Autodesk Fusion 360 part; units mm, degrees
(part 7 of 8)
  spline S19 degree 5 poles (-0.8149, 14.5372) (-0.8168, 14.5341) (-0.8204, 14.528) (-0.8258, 14.5188) (-0.833, 14.5066) (-0.842, 14.4913) (-0.8509, 14.4761) (-0.8597, 14.4608) (-0.8685, 14.4456) (-0.8773, 14.4304) (-0.886, 14.4152) (-0.8946, 14.4) (-0.9032, 14.3848) (-0.9117, 14.3697) (-0.9202, 14.3545) (-0.9286, 14.3394) (-0.937, 14.3243) (-0.9453, 14.3092) (-0.9536, 14.2941) (-0.9618, 14.2791) (-0.97, 14.264) (-0.9781, 14.249) (-0.9862, 14.234) (-0.9942, 14.219) (-1.0021, 14.204) (-1.01, 14.189) (-1.0179, 14.1741) (-1.0257, 14.1592) (-1.0334, 14.1443) (-1.0411, 14.1294) (-1.0488, 14.1145) (-1.0564, 14.0996) (-1.0639, 14.0848) (-1.0714, 14.07) (-1.0788, 14.0552) (-1.0862, 14.0404) (-1.0935, 14.0257) (-1.1008, 14.0109) (-1.108, 13.9962) (-1.1152, 13.9815) (-1.1223, 13.9669) (-1.1294, 13.9522) (-1.1364, 13.9376) (-1.1434, 13.923) (-1.1503, 13.9084) (-1.1572, 13.8938) (-1.164, 13.8793) (-1.1707, 13.8648) (-1.1775, 13.8503) (-1.1841, 13.8358) (-1.1907, 13.8214) (-1.1973, 13.807) (-1.2038, 13.7926) (-1.2102, 13.7782) (-1.2166, 13.7639) (-1.223, 13.7495) (-1.2293, 13.7352) (-1.2355, 13.721) (-1.2417, 13.7067) (-1.2478, 13.6925) (-1.2539, 13.6783) (-1.26, 13.6642) (-1.266, 13.65) (-1.2719, 13.6359) (-1.2778, 13.6218) (-1.2836, 13.6078) (-1.2894, 13.5938) (-1.2951, 13.5798) (-1.3008, 13.5658) (-1.3064, 13.5519) (-1.312, 13.538) (-1.3176, 13.5241) (-1.323, 13.5103) (-1.3285, 13.4964) (-1.3338, 13.4827) (-1.3392, 13.4689) (-1.3444, 13.4552) (-1.3497, 13.4415) (-1.3548, 13.4279) (-1.36, 13.4142) (-1.3651, 13.4006) (-1.3701, 13.3871) (-1.3751, 13.3736) (-1.38, 13.3601) (-1.3849, 13.3466) (-1.3897, 13.3332) (-1.3945, 13.3198) (-1.3992, 13.3065) (-1.4039, 13.2932) (-1.4085, 13.2799) (-1.4131, 13.2666) (-1.4176, 13.2534) (-1.4221, 13.2403) (-1.4265, 13.2271) (-1.4309, 13.214) (-1.4353, 13.201) (-1.4396, 13.188) (-1.4438, 13.175) (-1.448, 13.162) (-1.4521, 13.1491) (-1.4562, 13.1363) (-1.4603, 13.1235) (-1.4643, 13.1107) (-1.4682, 13.0979) (-1.4721, 13.0852) (-1.476, 13.0726) (-1.4798, 13.06) (-1.4835, 13.0474) (-1.4872, 13.0349) (-1.4909, 13.0224) (-1.4945, 13.01) (-1.4981, 12.9976) (-1.5016, 12.9852) (-1.5051, 12.9729) (-1.5085, 12.9606) (-1.5119, 12.9484) (-1.5152, 12.9362) (-1.5185, 12.9241) (-1.5218, 12.912) (-1.5249, 12.9) (-1.5281, 12.888) (-1.5312, 12.8761) (-1.5343, 12.8642) (-1.5373, 12.8524) (-1.5402, 12.8406) (-1.5432, 12.8288) (-1.546, 12.8171) (-1.5489, 12.8055) (-1.5517, 12.7939) (-1.5544, 12.7824) (-1.5571, 12.7709) (-1.5597, 12.7595) (-1.5624, 12.7481) (-1.5649, 12.7368) (-1.5674, 12.7255) (-1.5699, 12.7143) (-1.5723, 12.7031) (-1.5747, 12.692) (-1.5771, 12.681) (-1.5794, 12.67) (-1.5816, 12.659) (-1.5839, 12.6482) (-1.586, 12.6373) (-1.5882, 12.6266) (-1.5903, 12.6159) (-1.5923, 12.6052) (-1.5943, 12.5946) (-1.5963, 12.5841) (-1.5982, 12.5736) (-1.6001, 12.5632) (-1.6019, 12.5529) (-1.6037, 12.5426) (-1.6055, 12.5324) (-1.6072, 12.5223) (-1.6089, 12.5122) (-1.6105, 12.5022) (-1.6121, 12.4922) (-1.6137, 12.4823) (-1.6152, 12.4725) (-1.6167, 12.4627) (-1.6182, 12.453) (-1.6196, 12.4434) (-1.6209, 12.4339) (-1.6223, 12.4244) (-1.6236, 12.415) (-1.6248, 12.4056) (-1.626, 12.3964) (-1.6272, 12.3872) (-1.6284, 12.3781) (-1.6295, 12.369) (-1.6306, 12.36) (-1.6316, 12.3511) (-1.6326, 12.3423) (-1.6336, 12.3336) (-1.6345, 12.3249) (-1.6354, 12.3163) (-1.6363, 12.3078) (-1.6371, 12.2994) (-1.6379, 12.291) (-1.6387, 12.2827) (-1.6394, 12.2746) (-1.6401, 12.2665) (-1.6408, 12.2584) (-1.6414, 12.2505) (-1.6421, 12.2426) (-1.6426, 12.2349) (-1.6432, 12.2272) (-1.6437, 12.2196) (-1.6442, 12.2121) (-1.6447, 12.2047) (-1.6451, 12.1974) (-1.6455, 12.1901) (-1.6459, 12.183) (-1.6462, 12.1759) (-1.6466, 12.169) (-1.6469, 12.1621) (-1.6471, 12.1554) (-1.6474, 12.1487) (-1.6476, 12.1421) (-1.6478, 12.1357) (-1.648, 12.1293) (-1.6481, 12.123) (-1.6483, 12.1169) (-1.6484, 12.1108) (-1.6484, 12.1048) (-1.6485, 12.099) (-1.6486, 12.0933) (-1.6486, 12.0876) (-1.6486, 12.0821) (-1.6486, 12.0767) (-1.6486, 12.0714) (-1.6485, 12.0662) (-1.6485, 12.0611) (-1.6484, 12.0562) (-1.6483, 12.0514) (-1.6482, 12.0466) (-1.6481, 12.042) (-1.6479, 12.0376) (-1.6478, 12.0332) (-1.6476, 12.029) (-1.6475, 12.0249) (-1.6473, 12.021) (-1.6471, 12.0171) (-1.6469, 12.0134) (-1.6468, 12.0099) (-1.6466, 12.0064) (-1.6464, 12.0031) (-1.6462, 12) (-1.646, 11.997) (-1.6457, 11.9941) (-1.6455, 11.9914) (-1.6453, 11.9889) (-1.6451, 11.9865) (-1.6449, 11.9842) (-1.6448, 11.9821) (-1.6446, 11.9802) (-1.6444, 11.9784) (-1.6442, 11.9768) (-1.6441, 11.9753) (-1.6439, 11.974) (-1.6438, 11.9729) (-1.6437, 11.9722) (-1.6437, 11.9717) (-1.6436, 11.9714) (-1.6436, 11.9713) knots -1 -1 -1 -1 -1 -1 -0.99583333 -0.99166667 -0.9875 -0.98333333 -0.97916667 -0.975 -0.97083333 -0.96666667 -0.9625 -0.95833333 -0.95416667 -0.95 -0.94583333 -0.94166667 -0.9375 -0.93333333 -0.92916667 -0.925 -0.92083333 -0.91666667 -0.9125 -0.90833333 -0.90416667 -0.9 -0.89583333 -0.89166667 -0.8875 -0.88333333 -0.87916667 -0.875 -0.87083333 -0.86666667 -0.8625 -0.85833333 -0.85416667 -0.85 -0.84583333 -0.84166667 -0.8375 -0.83333333 -0.82916667 -0.825 -0.82083333 -0.81666667 -0.8125 -0.80833333 -0.80416667 -0.8 -0.79583333 -0.79166667 -0.7875 -0.78333333 -0.77916667 -0.775 -0.77083333 -0.76666667 -0.7625 -0.75833333 -0.75416667 -0.75 -0.74583333 -0.74166667 -0.7375 -0.73333333 -0.72916667 -0.725 -0.72083333 -0.71666667 -0.7125 -0.70833333 -0.70416667 -0.7 -0.69583333 -0.69166667 -0.6875 -0.68333333 -0.67916667 -0.675 -0.67083333 -0.66666667 -0.6625 -0.65833333 -0.65416667 -0.65 -0.64583333 -0.64166667 -0.6375 -0.63333333 -0.62916667 -0.625 -0.62083333 -0.61666667 -0.6125 -0.60833333 -0.60416667 -0.6 -0.59583333 -0.59166667 -0.5875 -0.58333333 -0.57916667 -0.575 -0.57083333 -0.56666667 -0.5625 -0.55833333 -0.55416667 -0.55 -0.54583333 -0.54166667 -0.5375 -0.53333333 -0.52916667 -0.525 -0.52083333 -0.51666667 -0.5125 -0.50833333 -0.50416667 -0.5 -0.49583333 -0.49166667 -0.4875 -0.48333333 -0.47916667 -0.475 -0.47083333 -0.46666667 -0.4625 -0.45833333 -0.45416667 -0.45 -0.44583333 -0.44166667 -0.4375 -0.43333333 -0.42916667 -0.425 -0.42083333 -0.41666667 -0.4125 -0.40833333 -0.40416667 -0.4 -0.39583333 -0.39166667 -0.3875 -0.38333333 -0.37916667 -0.375 -0.37083333 -0.36666667 -0.3625 -0.35833333 -0.35416667 -0.35 -0.34583333 -0.34166667 -0.3375 -0.33333333 -0.32916667 -0.325 -0.32083333 -0.31666667 -0.3125 -0.30833333 -0.30416667 -0.3 -0.29583333 -0.29166667 -0.2875 -0.28333333 -0.27916667 -0.275 -0.27083333 -0.26666667 -0.2625 -0.25833333 -0.25416667 -0.25 -0.24583333 -0.24166667 -0.2375 -0.23333333 -0.22916667 -0.225 -0.22083333 -0.21666667 -0.2125 -0.20833333 -0.20416667 -0.2 -0.19583333 -0.19166667 -0.1875 -0.18333333 -0.17916667 -0.175 -0.17083333 -0.16666667 -0.1625 -0.15833333 -0.15416667 -0.15 -0.14583333 -0.14166667 -0.1375 -0.13333333 -0.12916667 -0.125 -0.12083333 -0.11666667 -0.1125 -0.10833333 -0.10416667 -0.1 -0.09583333 -0.09166667 -0.0875 -0.08333333 -0.07916667 -0.075 -0.07083333 -0.06666667 -0.0625 -0.05833333 -0.05416667 -0.05 -0.04583333 -0.04166667 -0.0375 -0.03333333 -0.02916667 -0.025 -0.02083333 -0.01666667 -0.0125 -0.00833333 -0.00416667 0 0 0 0 0 0
  line L38 (-1.6436, 11.9713) -> (-1.6435, 11.9702)
  line L39 (-1.6435, 11.9702) -> (-1.3439, 9.7882)
  arc A20 (-1.3439, 9.7882) -> (-3.7302, 9.1488) centre (0, 0) ccw
  line L40 (-3.7302, 9.1488) -> (-4.5618, 11.1882)
  line L41 (-4.5618, 11.1882) -> (-4.5622, 11.1893)
  spline S20 degree 5 poles (-4.5622, 11.1893) (-4.5623, 11.1894) (-4.5624, 11.1897) (-4.5626, 11.1901) (-4.5629, 11.1908) (-4.5633, 11.1918) (-4.5638, 11.193) (-4.5644, 11.1943) (-4.5651, 11.1958) (-4.5658, 11.1974) (-4.5666, 11.1992) (-4.5675, 11.2011) (-4.5685, 11.2031) (-4.5695, 11.2053) (-4.5706, 11.2076) (-4.5718, 11.2101) (-4.5731, 11.2127) (-4.5744, 11.2154) (-4.5758, 11.2182) (-4.5773, 11.2212) (-4.5788, 11.2242) (-4.5804, 11.2274) (-4.5821, 11.2307) (-4.5839, 11.2341) (-4.5857, 11.2376) (-4.5876, 11.2413) (-4.5896, 11.245) (-4.5916, 11.2488) (-4.5938, 11.2528) (-4.596, 11.2568) (-4.5982, 11.2609) (-4.6006, 11.2652) (-4.603, 11.2695) (-4.6055, 11.2739) (-4.608, 11.2784) (-4.6106, 11.283) (-4.6133, 11.2877) (-4.6161, 11.2925) (-4.6189, 11.2973) (-4.6218, 11.3023) (-4.6248, 11.3073) (-4.6279, 11.3124) (-4.631, 11.3176) (-4.6342, 11.3229) (-4.6375, 11.3283) (-4.6408, 11.3337) (-4.6442, 11.3392) (-4.6477, 11.3448) (-4.6512, 11.3504) (-4.6548, 11.3561) (-4.6585, 11.3619) (-4.6623, 11.3678) (-4.6661, 11.3737) (-4.67, 11.3797) (-4.674, 11.3858) (-4.678, 11.3919) (-4.6821, 11.3981) (-4.6863, 11.4043) (-4.6906, 11.4106) (-4.6949, 11.417) (-4.6993, 11.4235) (-4.7037, 11.43) (-4.7082, 11.4365) (-4.7128, 11.4431) (-4.7175, 11.4498) (-4.7222, 11.4565) (-4.727, 11.4633) (-4.7319, 11.4701) (-4.7368, 11.477) (-4.7418, 11.484) (-4.7469, 11.4909) (-4.7521, 11.498) (-4.7573, 11.5051) (-4.7626, 11.5122) (-4.7679, 11.5194) (-4.7733, 11.5266) (-4.7788, 11.5339) (-4.7844, 11.5412) (-4.79, 11.5486) (-4.7957, 11.556) (-4.8014, 11.5635) (-4.8073, 11.571) (-4.8132, 11.5785) (-4.8191, 11.5861) (-4.8252, 11.5937) (-4.8312, 11.6014) (-4.8374, 11.6091) (-4.8436, 11.6168) (-4.8499, 11.6246) (-4.8563, 11.6325) (-4.8627, 11.6403) (-4.8692, 11.6482) (-4.8758, 11.6561) (-4.8824, 11.6641) (-4.8891, 11.6721) (-4.8959, 11.6801) (-4.9027, 11.6882) (-4.9096, 11.6963) (-4.9166, 11.7044) (-4.9236, 11.7126) (-4.9307, 11.7208) (-4.9379, 11.729) (-4.9451, 11.7373) (-4.9524, 11.7456) (-4.9598, 11.7539) (-4.9672, 11.7622) (-4.9747, 11.7706) (-4.9822, 11.779) (-4.9899, 11.7874) (-4.9976, 11.7958) (-5.0053, 11.8043) (-5.0131, 11.8128) (-5.021, 11.8213) (-5.029, 11.8299) (-5.037, 11.8385) (-5.045, 11.8471) (-5.0532, 11.8557) (-5.0614, 11.8643) (-5.0697, 11.873) (-5.078, 11.8817) (-5.0864, 11.8904) (-5.0949, 11.8991) (-5.1034, 11.9079) (-5.112, 11.9166) (-5.1206, 11.9254) (-5.1294, 11.9342) (-5.1381, 11.943) (-5.147, 11.9519) (-5.1559, 11.9607) (-5.1649, 11.9696) (-5.1739, 11.9785) (-5.183, 11.9874) (-5.1922, 11.9963) (-5.2014, 12.0053) (-5.2107, 12.0142) (-5.22, 12.0232) (-5.2295, 12.0322) (-5.2389, 12.0411) (-5.2485, 12.0502) (-5.2581, 12.0592) (-5.2677, 12.0682) (-5.2775, 12.0773) (-5.2873, 12.0863) (-5.2971, 12.0954) (-5.307, 12.1045) (-5.317, 12.1136) (-5.327, 12.1227) (-5.3371, 12.1318) (-5.3473, 12.1409) (-5.3575, 12.15) (-5.3678, 12.1592) (-5.3781, 12.1683) (-5.3885, 12.1775) (-5.399, 12.1866) (-5.4095, 12.1958) (-5.4201, 12.205) (-5.4308, 12.2141) (-5.4415, 12.2233) (-5.4523, 12.2325) (-5.4631, 12.2417) (-5.474, 12.2509) (-5.4849, 12.2602) (-5.4959, 12.2694) (-5.507, 12.2786) (-5.5181, 12.2878) (-5.5293, 12.2971) (-5.5406, 12.3063) (-5.5519, 12.3155) (-5.5633, 12.3248) (-5.5747, 12.334) (-5.5862, 12.3433) (-5.5977, 12.3525) (-5.6094, 12.3617) (-5.621, 12.371) (-5.6327, 12.3802) (-5.6445, 12.3895) (-5.6564, 12.3987) (-5.6683, 12.408) (-5.6802, 12.4172) (-5.6923, 12.4265) (-5.7043, 12.4358) (-5.7165, 12.445) (-5.7287, 12.4542) (-5.7409, 12.4635) (-5.7532, 12.4727) (-5.7656, 12.482) (-5.778, 12.4912) (-5.7905, 12.5005) (-5.8031, 12.5097) (-5.8157, 12.5189) (-5.8283, 12.5282) (-5.841, 12.5374) (-5.8538, 12.5466) (-5.8666, 12.5558) (-5.8795, 12.565) (-5.8924, 12.5742) (-5.9054, 12.5834) (-5.9185, 12.5926) (-5.9316, 12.6018) (-5.9448, 12.611) (-5.958, 12.6202) (-5.9713, 12.6294) (-5.9846, 12.6385) (-5.998, 12.6477) (-6.0115, 12.6568) (-6.025, 12.666) (-6.0385, 12.6751) (-6.0521, 12.6842) (-6.0658, 12.6934) (-6.0795, 12.7025) (-6.0933, 12.7116) (-6.1071, 12.7207) (-6.121, 12.7298) (-6.135, 12.7388) (-6.149, 12.7479) (-6.163, 12.757) (-6.1771, 12.766) (-6.1913, 12.775) (-6.2055, 12.7841) (-6.2198, 12.7931) (-6.2341, 12.8021) (-6.2485, 12.8111) (-6.2629, 12.8201) (-6.2774, 12.829) (-6.292, 12.838) (-6.3066, 12.847) (-6.3212, 12.8559) (-6.3359, 12.8648) (-6.3507, 12.8737) (-6.3655, 12.8826) (-6.3804, 12.8915) (-6.3953, 12.9004) (-6.4102, 12.9092) (-6.4253, 12.9181) (-6.4403, 12.9269) (-6.4555, 12.9357) (-6.4706, 12.9445) (-6.4859, 12.9533) (-6.5012, 12.9621) (-6.5165, 12.9708) (-6.5319, 12.9796) (-6.5442, 12.9866) (-6.5535, 12.9918) (-6.5597, 12.9953) (-6.5628, 12.997) knots 0 0 0 0 0 0 0.00416667 0.00833333 0.0125 0.01666667 0.02083333 0.025 0.02916667 0.03333333 0.0375 0.04166667 0.04583333 0.05 0.05416667 0.05833333 0.0625 0.06666667 0.07083333 0.075 0.07916667 0.08333333 0.0875 0.09166667 0.09583333 0.1 0.10416667 0.10833333 0.1125 0.11666667 0.12083333 0.125 0.12916667 0.13333333 0.1375 0.14166667 0.14583333 0.15 0.15416667 0.15833333 0.1625 0.16666667 0.17083333 0.175 0.17916667 0.18333333 0.1875 0.19166667 0.19583333 0.2 0.20416667 0.20833333 0.2125 0.21666667 0.22083333 0.225 0.22916667 0.23333333 0.2375 0.24166667 0.24583333 0.25 0.25416667 0.25833333 0.2625 0.26666667 0.27083333 0.275 0.27916667 0.28333333 0.2875 0.29166667 0.29583333 0.3 0.30416667 0.30833333 0.3125 0.31666667 0.32083333 0.325 0.32916667 0.33333333 0.3375 0.34166667 0.34583333 0.35 0.35416667 0.35833333 0.3625 0.36666667 0.37083333 0.375 0.37916667 0.38333333 0.3875 0.39166667 0.39583333 0.4 0.40416667 0.40833333 0.4125 0.41666667 0.42083333 0.425 0.42916667 0.43333333 0.4375 0.44166667 0.44583333 0.45 0.45416667 0.45833333 0.4625 0.46666667 0.47083333 0.475 0.47916667 0.48333333 0.4875 0.49166667 0.49583333 0.5 0.50416667 0.50833333 0.5125 0.51666667 0.52083333 0.525 0.52916667 0.53333333 0.5375 0.54166667 0.54583333 0.55 0.55416667 0.55833333 0.5625 0.56666667 0.57083333 0.575 0.57916667 0.58333333 0.5875 0.59166667 0.59583333 0.6 0.60416667 0.60833333 0.6125 0.61666667 0.62083333 0.625 0.62916667 0.63333333 0.6375 0.64166667 0.64583333 0.65 0.65416667 0.65833333 0.6625 0.66666667 0.67083333 0.675 0.67916667 0.68333333 0.6875 0.69166667 0.69583333 0.7 0.70416667 0.70833333 0.7125 0.71666667 0.72083333 0.725 0.72916667 0.73333333 0.7375 0.74166667 0.74583333 0.75 0.75416667 0.75833333 0.7625 0.76666667 0.77083333 0.775 0.77916667 0.78333333 0.7875 0.79166667 0.79583333 0.8 0.80416667 0.80833333 0.8125 0.81666667 0.82083333 0.825 0.82916667 0.83333333 0.8375 0.84166667 0.84583333 0.85 0.85416667 0.85833333 0.8625 0.86666667 0.87083333 0.875 0.87916667 0.88333333 0.8875 0.89166667 0.89583333 0.9 0.90416667 0.90833333 0.9125 0.91666667 0.92083333 0.925 0.92916667 0.93333333 0.9375 0.94166667 0.94583333 0.95 0.95416667 0.95833333 0.9625 0.96666667 0.97083333 0.975 0.97916667 0.98333333 0.9875 0.99166667 0.99583333 1 1 1 1 1 1
  arc A21 (-6.5628, 12.997) -> (-7.9743, 12.1821) centre (0, 0) ccw
  spline S21 degree 5 poles (-7.9743, 12.1821) (-7.9744, 12.1785) (-7.9745, 12.1714) (-7.9746, 12.1608) (-7.9747, 12.1466) (-7.9748, 12.1289) (-7.9749, 12.1112) (-7.975, 12.0936) (-7.975, 12.076) (-7.9749, 12.0585) (-7.9749, 12.041) (-7.9748, 12.0235) (-7.9746, 12.0061) (-7.9744, 11.9887) (-7.9742, 11.9713) (-7.9739, 11.954) (-7.9736, 11.9367) (-7.9733, 11.9195) (-7.9729, 11.9023) (-7.9725, 11.8851) (-7.972, 11.868) (-7.9716, 11.8509) (-7.971, 11.8339) (-7.9705, 11.8169) (-7.9699, 11.8) (-7.9692, 11.7831) (-7.9686, 11.7662) (-7.9679, 11.7494) (-7.9671, 11.7326) (-7.9663, 11.7158) (-7.9655, 11.6991) (-7.9647, 11.6825) (-7.9638, 11.6658) (-7.9629, 11.6493) (-7.9619, 11.6327) (-7.9609, 11.6163) (-7.9599, 11.5998) (-7.9588, 11.5834) (-7.9577, 11.5671) (-7.9566, 11.5508) (-7.9554, 11.5345) (-7.9542, 11.5183) (-7.953, 11.5021) (-7.9517, 11.486) (-7.9504, 11.4699) (-7.9491, 11.4538) (-7.9477, 11.4378) (-7.9463, 11.4219) (-7.9448, 11.406) (-7.9434, 11.3901) (-7.9419, 11.3743) (-7.9403, 11.3585) (-7.9388, 11.3428) (-7.9372, 11.3272) (-7.9355, 11.3115) (-7.9339, 11.296) (-7.9322, 11.2804) (-7.9305, 11.265) (-7.9287, 11.2495) (-7.9269, 11.2341) (-7.9251, 11.2188) (-7.9232, 11.2035) (-7.9214, 11.1883) (-7.9194, 11.1731) (-7.9175, 11.158) (-7.9155, 11.1429) (-7.9135, 11.1279) (-7.9115, 11.1129) (-7.9094, 11.0979) (-7.9074, 11.0831) (-7.9052, 11.0682) (-7.9031, 11.0534) (-7.9009, 11.0387) (-7.8987, 11.024) (-7.8965, 11.0094) (-7.8942, 10.9948) (-7.8919, 10.9803) (-7.8896, 10.9659) (-7.8873, 10.9514) (-7.8849, 10.9371) (-7.8825, 10.9228) (-7.8801, 10.9085) (-7.8776, 10.8943) (-7.8751, 10.8802) (-7.8726, 10.8661) (-7.8701, 10.852) (-7.8676, 10.8381) (-7.865, 10.8241) (-7.8624, 10.8103) (-7.8597, 10.7965) (-7.8571, 10.7827) (-7.8544, 10.769) (-7.8517, 10.7553) (-7.849, 10.7418) (-7.8462, 10.7282) (-7.8435, 10.7147) (-7.8407, 10.7013) (-7.8379, 10.688) (-7.835, 10.6747) (-7.8321, 10.6614) (-7.8293, 10.6482) (-7.8264, 10.6351) (-7.8234, 10.6221) (-7.8205, 10.609) (-7.8175, 10.5961) (-7.8145, 10.5832) (-7.8115, 10.5704) (-7.8085, 10.5576) (-7.8054, 10.5449) (-7.8024, 10.5323) (-7.7993, 10.5197) (-7.7962, 10.5072) (-7.793, 10.4947) (-7.7899, 10.4823) (-7.7867, 10.47) (-7.7835, 10.4577) (-7.7803, 10.4455) (-7.7771, 10.4334) (-7.7739, 10.4213) (-7.7706, 10.4093) (-7.7674, 10.3973) (-7.7641, 10.3854) (-7.7608, 10.3736) (-7.7575, 10.3618) (-7.7542, 10.3501) (-7.7508, 10.3385) (-7.7475, 10.327) (-7.7441, 10.3155) (-7.7407, 10.304) (-7.7373, 10.2927) (-7.7339, 10.2814) (-7.7305, 10.2702) (-7.7271, 10.259) (-7.7236, 10.2479) (-7.7202, 10.2369) (-7.7167, 10.2259) (-7.7133, 10.215) (-7.7098, 10.2042) (-7.7063, 10.1935) (-7.7028, 10.1828) (-7.6993, 10.1722) (-7.6957, 10.1617) (-7.6922, 10.1512) (-7.6887, 10.1408) (-7.6851, 10.1305) (-7.6816, 10.1203) (-7.678, 10.1101) (-7.6745, 10.1) (-7.6709, 10.09) (-7.6673, 10.08) (-7.6638, 10.0702) (-7.6602, 10.0604) (-7.6566, 10.0506) (-7.653, 10.041) (-7.6494, 10.0314) (-7.6458, 10.0219) (-7.6423, 10.0125) (-7.6387, 10.0031) (-7.6351, 9.9939) (-7.6315, 9.9847) (-7.6279, 9.9756) (-7.6243, 9.9665) (-7.6207, 9.9576) (-7.6171, 9.9487) (-7.6135, 9.9399) (-7.61, 9.9312) (-7.6064, 9.9226) (-7.6028, 9.914) (-7.5992, 9.9055) (-7.5957, 9.8971) (-7.5921, 9.8888) (-7.5886, 9.8806) (-7.585, 9.8725) (-7.5815, 9.8644) (-7.578, 9.8564) (-7.5745, 9.8485) (-7.571, 9.8407) (-7.5675, 9.833) (-7.564, 9.8254) (-7.5605, 9.8178) (-7.5571, 9.8104) (-7.5536, 9.803) (-7.5502, 9.7957) (-7.5468, 9.7885) (-7.5434, 9.7814) (-7.54, 9.7744) (-7.5366, 9.7675) (-7.5333, 9.7606) (-7.53, 9.7539) (-7.5267, 9.7472) (-7.5234, 9.7407) (-7.5201, 9.7342) (-7.5169, 9.7278) (-7.5136, 9.7215) (-7.5104, 9.7154) (-7.5073, 9.7093) (-7.5041, 9.7033) (-7.501, 9.6974) (-7.4979, 9.6916) (-7.4949, 9.6859) (-7.4918, 9.6803) (-7.4888, 9.6748) (-7.4859, 9.6694) (-7.4829, 9.6641) (-7.48, 9.6589) (-7.4772, 9.6538) (-7.4743, 9.6488) (-7.4715, 9.6439) (-7.4688, 9.6391) (-7.4661, 9.6344) (-7.4634, 9.6299) (-7.4608, 9.6254) (-7.4582, 9.621) (-7.4556, 9.6168) (-7.4531, 9.6126) (-7.4507, 9.6086) (-7.4483, 9.6047) (-7.4459, 9.6009) (-7.4436, 9.5972) (-7.4414, 9.5936) (-7.4392, 9.5901) (-7.4371, 9.5868) (-7.435, 9.5836) (-7.433, 9.5805) (-7.4311, 9.5775) (-7.4292, 9.5746) (-7.4274, 9.5719) (-7.4256, 9.5692) (-7.4239, 9.5667) (-7.4223, 9.5644) (-7.4208, 9.5621) (-7.4193, 9.56) (-7.418, 9.558) (-7.4167, 9.5561) (-7.4154, 9.5544) (-7.4143, 9.5528) (-7.4133, 9.5514) (-7.4123, 9.5501) (-7.4115, 9.5489) (-7.4107, 9.5479) (-7.4101, 9.547) (-7.4096, 9.5464) (-7.4093, 9.546) (-7.4092, 9.5458) (-7.4091, 9.5457) knots -1 -1 -1 -1 -1 -1 -0.99583333 -0.99166667 -0.9875 -0.98333333 -0.97916667 -0.975 -0.97083333 -0.96666667 -0.9625 -0.95833333 -0.95416667 -0.95 -0.94583333 -0.94166667 -0.9375 -0.93333333 -0.92916667 -0.925 -0.92083333 -0.91666667 -0.9125 -0.90833333 -0.90416667 -0.9 -0.89583333 -0.89166667 -0.8875 -0.88333333 -0.87916667 -0.875 -0.87083333 -0.86666667 -0.8625 -0.85833333 -0.85416667 -0.85 -0.84583333 -0.84166667 -0.8375 -0.83333333 -0.82916667 -0.825 -0.82083333 -0.81666667 -0.8125 -0.80833333 -0.80416667 -0.8 -0.79583333 -0.79166667 -0.7875 -0.78333333 -0.77916667 -0.775 -0.77083333 -0.76666667 -0.7625 -0.75833333 -0.75416667 -0.75 -0.74583333 -0.74166667 -0.7375 -0.73333333 -0.72916667 -0.725 -0.72083333 -0.71666667 -0.7125 -0.70833333 -0.70416667 -0.7 -0.69583333 -0.69166667 -0.6875 -0.68333333 -0.67916667 -0.675 -0.67083333 -0.66666667 -0.6625 -0.65833333 -0.65416667 -0.65 -0.64583333 -0.64166667 -0.6375 -0.63333333 -0.62916667 -0.625 -0.62083333 -0.61666667 -0.6125 -0.60833333 -0.60416667 -0.6 -0.59583333 -0.59166667 -0.5875 -0.58333333 -0.57916667 -0.575 -0.57083333 -0.56666667 -0.5625 -0.55833333 -0.55416667 -0.55 -0.54583333 -0.54166667 -0.5375 -0.53333333 -0.52916667 -0.525 -0.52083333 -0.51666667 -0.5125 -0.50833333 -0.50416667 -0.5 -0.49583333 -0.49166667 -0.4875 -0.48333333 -0.47916667 -0.475 -0.47083333 -0.46666667 -0.4625 -0.45833333 -0.45416667 -0.45 -0.44583333 -0.44166667 -0.4375 -0.43333333 -0.42916667 -0.425 -0.42083333 -0.41666667 -0.4125 -0.40833333 -0.40416667 -0.4 -0.39583333 -0.39166667 -0.3875 -0.38333333 -0.37916667 -0.375 -0.37083333 -0.36666667 -0.3625 -0.35833333 -0.35416667 -0.35 -0.34583333 -0.34166667 -0.3375 -0.33333333 -0.32916667 -0.325 -0.32083333 -0.31666667 -0.3125 -0.30833333 -0.30416667 -0.3 -0.29583333 -0.29166667 -0.2875 -0.28333333 -0.27916667 -0.275 -0.27083333 -0.26666667 -0.2625 -0.25833333 -0.25416667 -0.25 -0.24583333 -0.24166667 -0.2375 -0.23333333 -0.22916667 -0.225 -0.22083333 -0.21666667 -0.2125 -0.20833333 -0.20416667 -0.2 -0.19583333 -0.19166667 -0.1875 -0.18333333 -0.17916667 -0.175 -0.17083333 -0.16666667 -0.1625 -0.15833333 -0.15416667 -0.15 -0.14583333 -0.14166667 -0.1375 -0.13333333 -0.12916667 -0.125 -0.12083333 -0.11666667 -0.1125 -0.10833333 -0.10416667 -0.1 -0.09583333 -0.09166667 -0.0875 -0.08333333 -0.07916667 -0.075 -0.07083333 -0.06666667 -0.0625 -0.05833333 -0.05416667 -0.05 -0.04583333 -0.04166667 -0.0375 -0.03333333 -0.02916667 -0.025 -0.02083333 -0.01666667 -0.0125 -0.00833333 -0.00416667 0 0 0 0 0 0
  line L42 (-7.4091, 9.5457) -> (-7.4084, 9.5447)
  line L43 (-7.4084, 9.5447) -> (-6.0579, 7.8049)
  arc A22 (-6.0579, 7.8049) -> (-7.8049, 6.0579) centre (0, 0) ccw
  line L44 (-7.8049, 6.0579) -> (-9.5447, 7.4084)
  line L45 (-9.5447, 7.4084) -> (-9.5457, 7.4091)
  spline S22 degree 5 poles (-9.5457, 7.4091) (-9.5458, 7.4092) (-9.546, 7.4093) (-9.5464, 7.4096) (-9.547, 7.4101) (-9.5479, 7.4107) (-9.5489, 7.4115) (-9.5501, 7.4123) (-9.5514, 7.4133) (-9.5528, 7.4143) (-9.5544, 7.4154) (-9.5561, 7.4167) (-9.558, 7.418) (-9.56, 7.4193) (-9.5621, 7.4208) (-9.5644, 7.4223) (-9.5667, 7.4239) (-9.5692, 7.4256) (-9.5719, 7.4274) (-9.5746, 7.4292) (-9.5775, 7.4311) (-9.5805, 7.433) (-9.5836, 7.435) (-9.5868, 7.4371) (-9.5901, 7.4392) (-9.5936, 7.4414) (-9.5972, 7.4436) (-9.6009, 7.4459) (-9.6047, 7.4483) (-9.6086, 7.4507) (-9.6126, 7.4531) (-9.6168, 7.4556) (-9.621, 7.4582) (-9.6254, 7.4608) (-9.6299, 7.4634) (-9.6344, 7.4661) (-9.6391, 7.4688) (-9.6439, 7.4715) (-9.6488, 7.4743) (-9.6538, 7.4772) (-9.6589, 7.48) (-9.6641, 7.4829) (-9.6694, 7.4859) (-9.6748, 7.4888) (-9.6803, 7.4918) (-9.6859, 7.4949) (-9.6916, 7.4979) (-9.6974, 7.501) (-9.7033, 7.5041) (-9.7093, 7.5073) (-9.7154, 7.5104) (-9.7215, 7.5136) (-9.7278, 7.5169) (-9.7342, 7.5201) (-9.7407, 7.5234) (-9.7472, 7.5267) (-9.7539, 7.53) (-9.7606, 7.5333) (-9.7675, 7.5366) (-9.7744, 7.54) (-9.7814, 7.5434) (-9.7885, 7.5468) (-9.7957, 7.5502) (-9.803, 7.5536) (-9.8104, 7.5571) (-9.8178, 7.5605) (-9.8254, 7.564) (-9.833, 7.5675) (-9.8407, 7.571) (-9.8485, 7.5745) (-9.8564, 7.578) (-9.8644, 7.5815) (-9.8725, 7.585) (-9.8806, 7.5886) (-9.8888, 7.5921) (-9.8971, 7.5957) (-9.9055, 7.5992) (-9.914, 7.6028) (-9.9226, 7.6064) (-9.9312, 7.61) (-9.9399, 7.6135) (-9.9487, 7.6171) (-9.9576, 7.6207) (-9.9665, 7.6243) (-9.9756, 7.6279) (-9.9847, 7.6315) (-9.9939, 7.6351) (-10.0031, 7.6387) (-10.0125, 7.6423) (-10.0219, 7.6458) (-10.0314, 7.6494) (-10.041, 7.653) (-10.0506, 7.6566) (-10.0604, 7.6602) (-10.0702, 7.6638) (-10.08, 7.6673) (-10.09, 7.6709) (-10.1, 7.6745) (-10.1101, 7.678) (-10.1203, 7.6816) (-10.1305, 7.6851) (-10.1408, 7.6887) (-10.1512, 7.6922) (-10.1617, 7.6957) (-10.1722, 7.6993) (-10.1828, 7.7028) (-10.1935, 7.7063) (-10.2042, 7.7098) (-10.215, 7.7133) (-10.2259, 7.7167) (-10.2369, 7.7202) (-10.2479, 7.7236) (-10.259, 7.7271) (-10.2702, 7.7305) (-10.2814, 7.7339) (-10.2927, 7.7373) (-10.304, 7.7407) (-10.3155, 7.7441) (-10.327, 7.7475) (-10.3385, 7.7508) (-10.3501, 7.7542) (-10.3618, 7.7575) (-10.3736, 7.7608) (-10.3854, 7.7641) (-10.3973, 7.7674) (-10.4093, 7.7706) (-10.4213, 7.7739) (-10.4334, 7.7771) (-10.4455, 7.7803) (-10.4577, 7.7835) (-10.47, 7.7867) (-10.4823, 7.7899) (-10.4947, 7.793) (-10.5072, 7.7962) (-10.5197, 7.7993) (-10.5323, 7.8024) (-10.5449, 7.8054) (-10.5576, 7.8085) (-10.5704, 7.8115) (-10.5832, 7.8145) (-10.5961, 7.8175) (-10.609, 7.8205) (-10.6221, 7.8234) (-10.6351, 7.8264) (-10.6482, 7.8293) (-10.6614, 7.8321) (-10.6747, 7.835) (-10.688, 7.8379) (-10.7013, 7.8407) (-10.7147, 7.8435) (-10.7282, 7.8462) (-10.7418, 7.849) (-10.7553, 7.8517) (-10.769, 7.8544) (-10.7827, 7.8571) (-10.7965, 7.8597) (-10.8103, 7.8624) (-10.8241, 7.865) (-10.8381, 7.8676) (-10.852, 7.8701) (-10.8661, 7.8726) (-10.8802, 7.8751) (-10.8943, 7.8776) (-10.9085, 7.8801) (-10.9228, 7.8825) (-10.9371, 7.8849) (-10.9514, 7.8873) (-10.9659, 7.8896) (-10.9803, 7.8919) (-10.9948, 7.8942) (-11.0094, 7.8965) (-11.024, 7.8987) (-11.0387, 7.9009) (-11.0534, 7.9031) (-11.0682, 7.9052) (-11.0831, 7.9074) (-11.0979, 7.9094) (-11.1129, 7.9115) (-11.1279, 7.9135) (-11.1429, 7.9155) (-11.158, 7.9175) (-11.1731, 7.9194) (-11.1883, 7.9214) (-11.2035, 7.9232) (-11.2188, 7.9251) (-11.2341, 7.9269) (-11.2495, 7.9287) (-11.265, 7.9305) (-11.2804, 7.9322) (-11.296, 7.9339) (-11.3115, 7.9355) (-11.3272, 7.9372) (-11.3428, 7.9388) (-11.3585, 7.9403) (-11.3743, 7.9419) (-11.3901, 7.9434) (-11.406, 7.9448) (-11.4219, 7.9463) (-11.4378, 7.9477) (-11.4538, 7.9491) (-11.4699, 7.9504) (-11.486, 7.9517) (-11.5021, 7.953) (-11.5183, 7.9542) (-11.5345, 7.9554) (-11.5508, 7.9566) (-11.5671, 7.9577) (-11.5834, 7.9588) (-11.5998, 7.9599) (-11.6163, 7.9609) (-11.6327, 7.9619) (-11.6493, 7.9629) (-11.6658, 7.9638) (-11.6825, 7.9647) (-11.6991, 7.9655) (-11.7158, 7.9663) (-11.7326, 7.9671) (-11.7494, 7.9679) (-11.7662, 7.9686) (-11.7831, 7.9692) (-11.8, 7.9699) (-11.8169, 7.9705) (-11.8339, 7.971) (-11.8509, 7.9716) (-11.868, 7.972) (-11.8851, 7.9725) (-11.9023, 7.9729) (-11.9195, 7.9733) (-11.9367, 7.9736) (-11.954, 7.9739) (-11.9713, 7.9742) (-11.9887, 7.9744) (-12.0061, 7.9746) (-12.0235, 7.9748) (-12.041, 7.9749) (-12.0585, 7.9749) (-12.076, 7.975) (-12.0936, 7.975) (-12.1112, 7.9749) (-12.1289, 7.9748) (-12.1466, 7.9747) (-12.1608, 7.9746) (-12.1714, 7.9745) (-12.1785, 7.9744) (-12.1821, 7.9743) knots 0 0 0 0 0 0 0.00416667 0.00833333 0.0125 0.01666667 0.02083333 0.025 0.02916667 0.03333333 0.0375 0.04166667 0.04583333 0.05 0.05416667 0.05833333 0.0625 0.06666667 0.07083333 0.075 0.07916667 0.08333333 0.0875 0.09166667 0.09583333 0.1 0.10416667 0.10833333 0.1125 0.11666667 0.12083333 0.125 0.12916667 0.13333333 0.1375 0.14166667 0.14583333 0.15 0.15416667 0.15833333 0.1625 0.16666667 0.17083333 0.175 0.17916667 0.18333333 0.1875 0.19166667 0.19583333 0.2 0.20416667 0.20833333 0.2125 0.21666667 0.22083333 0.225 0.22916667 0.23333333 0.2375 0.24166667 0.24583333 0.25 0.25416667 0.25833333 0.2625 0.26666667 0.27083333 0.275 0.27916667 0.28333333 0.2875 0.29166667 0.29583333 0.3 0.30416667 0.30833333 0.3125 0.31666667 0.32083333 0.325 0.32916667 0.33333333 0.3375 0.34166667 0.34583333 0.35 0.35416667 0.35833333 0.3625 0.36666667 0.37083333 0.375 0.37916667 0.38333333 0.3875 0.39166667 0.39583333 0.4 0.40416667 0.40833333 0.4125 0.41666667 0.42083333 0.425 0.42916667 0.43333333 0.4375 0.44166667 0.44583333 0.45 0.45416667 0.45833333 0.4625 0.46666667 0.47083333 0.475 0.47916667 0.48333333 0.4875 0.49166667 0.49583333 0.5 0.50416667 0.50833333 0.5125 0.51666667 0.52083333 0.525 0.52916667 0.53333333 0.5375 0.54166667 0.54583333 0.55 0.55416667 0.55833333 0.5625 0.56666667 0.57083333 0.575 0.57916667 0.58333333 0.5875 0.59166667 0.59583333 0.6 0.60416667 0.60833333 0.6125 0.61666667 0.62083333 0.625 0.62916667 0.63333333 0.6375 0.64166667 0.64583333 0.65 0.65416667 0.65833333 0.6625 0.66666667 0.67083333 0.675 0.67916667 0.68333333 0.6875 0.69166667 0.69583333 0.7 0.70416667 0.70833333 0.7125 0.71666667 0.72083333 0.725 0.72916667 0.73333333 0.7375 0.74166667 0.74583333 0.75 0.75416667 0.75833333 0.7625 0.76666667 0.77083333 0.775 0.77916667 0.78333333 0.7875 0.79166667 0.79583333 0.8 0.80416667 0.80833333 0.8125 0.81666667 0.82083333 0.825 0.82916667 0.83333333 0.8375 0.84166667 0.84583333 0.85 0.85416667 0.85833333 0.8625 0.86666667 0.87083333 0.875 0.87916667 0.88333333 0.8875 0.89166667 0.89583333 0.9 0.90416667 0.90833333 0.9125 0.91666667 0.92083333 0.925 0.92916667 0.93333333 0.9375 0.94166667 0.94583333 0.95 0.95416667 0.95833333 0.9625 0.96666667 0.97083333 0.975 0.97916667 0.98333333 0.9875 0.99166667 0.99583333 1 1 1 1 1 1
  arc A23 (-12.1821, 7.9743) -> (-12.997, 6.5628) centre (0, 0) ccw
  spline S23 degree 5 poles (-12.997, 6.5628) (-12.9953, 6.5597) (-12.9918, 6.5535) (-12.9866, 6.5442) (-12.9796, 6.5319) (-12.9708, 6.5165) (-12.9621, 6.5012) (-12.9533, 6.4859) (-12.9445, 6.4706) (-12.9357, 6.4555) (-12.9269, 6.4403) (-12.9181, 6.4253) (-12.9092, 6.4102) (-12.9004, 6.3953) (-12.8915, 6.3804) (-12.8826, 6.3655) (-12.8737, 6.3507) (-12.8648, 6.3359) (-12.8559, 6.3212) (-12.847, 6.3066) (-12.838, 6.292) (-12.829, 6.2774) (-12.8201, 6.2629) (-12.8111, 6.2485) (-12.8021, 6.2341) (-12.7931, 6.2198) (-12.7841, 6.2055) (-12.775, 6.1913) (-12.766, 6.1771) (-12.757, 6.163) (-12.7479, 6.149) (-12.7388, 6.135) (-12.7298, 6.121) (-12.7207, 6.1071) (-12.7116, 6.0933) (-12.7025, 6.0795) (-12.6934, 6.0658) (-12.6842, 6.0521) (-12.6751, 6.0385) (-12.666, 6.025) (-12.6568, 6.0115) (-12.6477, 5.998) (-12.6385, 5.9846) (-12.6294, 5.9713) (-12.6202, 5.958) (-12.611, 5.9448) (-12.6018, 5.9316) (-12.5926, 5.9185) (-12.5834, 5.9054) (-12.5742, 5.8924) (-12.565, 5.8795) (-12.5558, 5.8666) (-12.5466, 5.8538) (-12.5374, 5.841) (-12.5282, 5.8283) (-12.5189, 5.8157) (-12.5097, 5.8031) (-12.5005, 5.7905) (-12.4912, 5.778) (-12.482, 5.7656) (-12.4727, 5.7532) (-12.4635, 5.7409) (-12.4542, 5.7287) (-12.445, 5.7165) (-12.4358, 5.7043) (-12.4265, 5.6923) (-12.4172, 5.6802) (-12.408, 5.6683) (-12.3987, 5.6564) (-12.3895, 5.6445) (-12.3802, 5.6327) (-12.371, 5.621) (-12.3617, 5.6094) (-12.3525, 5.5977) (-12.3433, 5.5862) (-12.334, 5.5747) (-12.3248, 5.5633) (-12.3155, 5.5519) (-12.3063, 5.5406) (-12.2971, 5.5293) (-12.2878, 5.5181) (-12.2786, 5.507) (-12.2694, 5.4959) (-12.2602, 5.4849) (-12.2509, 5.474) (-12.2417, 5.4631) (-12.2325, 5.4523) (-12.2233, 5.4415) (-12.2141, 5.4308) (-12.205, 5.4201) (-12.1958, 5.4095) (-12.1866, 5.399) (-12.1775, 5.3885) (-12.1683, 5.3781) (-12.1592, 5.3678) (-12.15, 5.3575) (-12.1409, 5.3473) (-12.1318, 5.3371) (-12.1227, 5.327) (-12.1136, 5.317) (-12.1045, 5.307) (-12.0954, 5.2971) (-12.0863, 5.2873) (-12.0773, 5.2775) (-12.0682, 5.2677) (-12.0592, 5.2581) (-12.0502, 5.2485) (-12.0411, 5.2389) (-12.0322, 5.2295) (-12.0232, 5.22) (-12.0142, 5.2107) (-12.0053, 5.2014) (-11.9963, 5.1922) (-11.9874, 5.183) (-11.9785, 5.1739) (-11.9696, 5.1649) (-11.9607, 5.1559) (-11.9519, 5.147) (-11.943, 5.1381) (-11.9342, 5.1294) (-11.9254, 5.1206) (-11.9166, 5.112) (-11.9079, 5.1034) (-11.8991, 5.0949) (-11.8904, 5.0864) (-11.8817, 5.078) (-11.873, 5.0697) (-11.8643, 5.0614) (-11.8557, 5.0532) (-11.8471, 5.045) (-11.8385, 5.037) (-11.8299, 5.029) (-11.8213, 5.021) (-11.8128, 5.0131) (-11.8043, 5.0053) (-11.7958, 4.9976) (-11.7874, 4.9899) (-11.779, 4.9822) (-11.7706, 4.9747) (-11.7622, 4.9672) (-11.7539, 4.9598) (-11.7456, 4.9524) (-11.7373, 4.9451) (-11.729, 4.9379) (-11.7208, 4.9307) (-11.7126, 4.9236) (-11.7044, 4.9166) (-11.6963, 4.9096) (-11.6882, 4.9027) (-11.6801, 4.8959) (-11.6721, 4.8891) (-11.6641, 4.8824) (-11.6561, 4.8758) (-11.6482, 4.8692) (-11.6403, 4.8627) (-11.6325, 4.8563) (-11.6246, 4.8499) (-11.6168, 4.8436) (-11.6091, 4.8374) (-11.6014, 4.8312) (-11.5937, 4.8252) (-11.5861, 4.8191) (-11.5785, 4.8132) (-11.571, 4.8073) (-11.5635, 4.8014) (-11.556, 4.7957) (-11.5486, 4.79) (-11.5412, 4.7844) (-11.5339, 4.7788) (-11.5266, 4.7733) (-11.5194, 4.7679) (-11.5122, 4.7626) (-11.5051, 4.7573) (-11.498, 4.7521) (-11.4909, 4.7469) (-11.484, 4.7418) (-11.477, 4.7368) (-11.4701, 4.7319) (-11.4633, 4.727) (-11.4565, 4.7222) (-11.4498, 4.7175) (-11.4431, 4.7128) (-11.4365, 4.7082) (-11.43, 4.7037) (-11.4235, 4.6993) (-11.417, 4.6949) (-11.4106, 4.6906) (-11.4043, 4.6863) (-11.3981, 4.6821) (-11.3919, 4.678) (-11.3858, 4.674) (-11.3797, 4.67) (-11.3737, 4.6661) (-11.3678, 4.6623) (-11.3619, 4.6585) (-11.3561, 4.6548) (-11.3504, 4.6512) (-11.3448, 4.6477) (-11.3392, 4.6442) (-11.3337, 4.6408) (-11.3283, 4.6375) (-11.3229, 4.6342) (-11.3176, 4.631) (-11.3124, 4.6279) (-11.3073, 4.6248) (-11.3023, 4.6218) (-11.2973, 4.6189) (-11.2925, 4.6161) (-11.2877, 4.6133) (-11.283, 4.6106) (-11.2784, 4.608) (-11.2739, 4.6055) (-11.2695, 4.603) (-11.2652, 4.6006) (-11.2609, 4.5982) (-11.2568, 4.596) (-11.2528, 4.5938) (-11.2488, 4.5916) (-11.245, 4.5896) (-11.2413, 4.5876) (-11.2376, 4.5857) (-11.2341, 4.5839) (-11.2307, 4.5821) (-11.2274, 4.5804) (-11.2242, 4.5788) (-11.2212, 4.5773) (-11.2182, 4.5758) (-11.2154, 4.5744) (-11.2127, 4.5731) (-11.2101, 4.5718) (-11.2076, 4.5706) (-11.2053, 4.5695) (-11.2031, 4.5685) (-11.2011, 4.5675) (-11.1992, 4.5666) (-11.1974, 4.5658) (-11.1958, 4.5651) (-11.1943, 4.5644) (-11.193, 4.5638) (-11.1918, 4.5633) (-11.1908, 4.5629) (-11.1901, 4.5626) (-11.1897, 4.5624) (-11.1894, 4.5623) (-11.1893, 4.5622) knots -1 -1 -1 -1 -1 -1 -0.99583333 -0.99166667 -0.9875 -0.98333333 -0.97916667 -0.975 -0.97083333 -0.96666667 -0.9625 -0.95833333 -0.95416667 -0.95 -0.94583333 -0.94166667 -0.9375 -0.93333333 -0.92916667 -0.925 -0.92083333 -0.91666667 -0.9125 -0.90833333 -0.90416667 -0.9 -0.89583333 -0.89166667 -0.8875 -0.88333333 -0.87916667 -0.875 -0.87083333 -0.86666667 -0.8625 -0.85833333 -0.85416667 -0.85 -0.84583333 -0.84166667 -0.8375 -0.83333333 -0.82916667 -0.825 -0.82083333 -0.81666667 -0.8125 -0.80833333 -0.80416667 -0.8 -0.79583333 -0.79166667 -0.7875 -0.78333333 -0.77916667 -0.775 -0.77083333 -0.76666667 -0.7625 -0.75833333 -0.75416667 -0.75 -0.74583333 -0.74166667 -0.7375 -0.73333333 -0.72916667 -0.725 -0.72083333 -0.71666667 -0.7125 -0.70833333 -0.70416667 -0.7 -0.69583333 -0.69166667 -0.6875 -0.68333333 -0.67916667 -0.675 -0.67083333 -0.66666667 -0.6625 -0.65833333 -0.65416667 -0.65 -0.64583333 -0.64166667 -0.6375 -0.63333333 -0.62916667 -0.625 -0.62083333 -0.61666667 -0.6125 -0.60833333 -0.60416667 -0.6 -0.59583333 -0.59166667 -0.5875 -0.58333333 -0.57916667 -0.575 -0.57083333 -0.56666667 -0.5625 -0.55833333 -0.55416667 -0.55 -0.54583333 -0.54166667 -0.5375 -0.53333333 -0.52916667 -0.525 -0.52083333 -0.51666667 -0.5125 -0.50833333 -0.50416667 -0.5 -0.49583333 -0.49166667 -0.4875 -0.48333333 -0.47916667 -0.475 -0.47083333 -0.46666667 -0.4625 -0.45833333 -0.45416667 -0.45 -0.44583333 -0.44166667 -0.4375 -0.43333333 -0.42916667 -0.425 -0.42083333 -0.41666667 -0.4125 -0.40833333 -0.40416667 -0.4 -0.39583333 -0.39166667 -0.3875 -0.38333333 -0.37916667 -0.375 -0.37083333 -0.36666667 -0.3625 -0.35833333 -0.35416667 -0.35 -0.34583333 -0.34166667 -0.3375 -0.33333333 -0.32916667 -0.325 -0.32083333 -0.31666667 -0.3125 -0.30833333 -0.30416667 -0.3 -0.29583333 -0.29166667 -0.2875 -0.28333333 -0.27916667 -0.275 -0.27083333 -0.26666667 -0.2625 -0.25833333 -0.25416667 -0.25 -0.24583333 -0.24166667 -0.2375 -0.23333333 -0.22916667 -0.225 -0.22083333 -0.21666667 -0.2125 -0.20833333 -0.20416667 -0.2 -0.19583333 -0.19166667 -0.1875 -0.18333333 -0.17916667 -0.175 -0.17083333 -0.16666667 -0.1625 -0.15833333 -0.15416667 -0.15 -0.14583333 -0.14166667 -0.1375 -0.13333333 -0.12916667 -0.125 -0.12083333 -0.11666667 -0.1125 -0.10833333 -0.10416667 -0.1 -0.09583333 -0.09166667 -0.0875 -0.08333333 -0.07916667 -0.075 -0.07083333 -0.06666667 -0.0625 -0.05833333 -0.05416667 -0.05 -0.04583333 -0.04166667 -0.0375 -0.03333333 -0.02916667 -0.025 -0.02083333 -0.01666667 -0.0125 -0.00833333 -0.00416667 0 0 0 0 0 0
  line L46 (-11.1893, 4.5622) -> (-11.1882, 4.5618)
  line L47 (-11.1882, 4.5618) -> (-9.1488, 3.7302)
  line L48 (0, 0) -> (0, -7.38)
  circle A24 centre (0, -7.38) radius 0.95
  line L49 (0, 0) -> (7.38, 0)
  line L50 (0, 0) -> (-7.38, 0)
  line L51 (0, 0) -> (0, 7.38)
  circle A25 centre (7.38, 0) radius 0.95
  circle A26 centre (0, 7.38) radius 0.95
  circle A27 centre (-7.38, 0) radius 0.95
  dimension "d7" = 7.38
  dimension "d8" = 1.9
  dimension "d9" = 7.38
  dimension "d10" = 7.38
  dimension "d11" = 7.38
  dimension "d12" = 1.9
  dimension "d13" = 1.9
  dimension "d14" = 1.9
  constraint coincident A0.centre A1.centre
  constraint vertical L48
  constraint coincident L48.end A24.centre
  constraint perpendicular L48 L49
  constraint perpendicular L48 L50
  constraint perpendicular L49 L51
  constraint coincident L49.end A25.centre
  constraint coincident L51.end A26.centre
  constraint coincident L50.end A27.centre
  measures "d7" distance of A0.centre L48.end
  measures "d8" diameter of A24
  measures "d9" distance of A0.centre L49.end
  measures "d10" distance of A0.centre L50.end
  measures "d11" distance of A0.centre L51.end
  measures "d12" diameter of A25
  measures "d13" diameter of A26
  measures "d14" diameter of A27